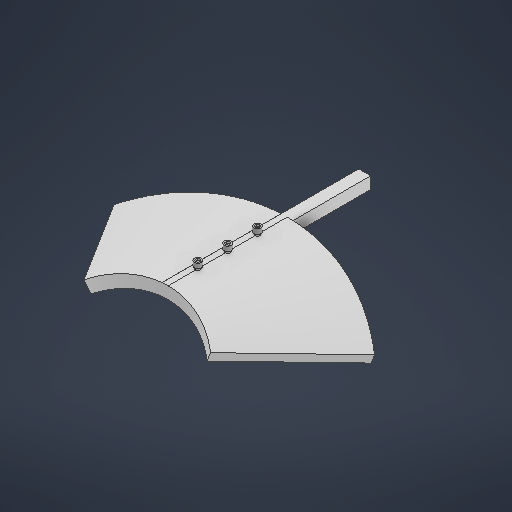
# Autodesk Inventor part: rod
Saved by Autodesk Inventor 2026.2 (Build 302298000, 298)
## iProperties
Created: 2025-12-16
Part Number: rod
Material: Generic
Document SubType Name: Modeling
Designer: Thoma
Density: 1 g/cm^3
Appearance: Default
Author: Thoma
Autodesk Inventor part; units mm, degrees
ref_plane "YZ Plane" through (0, 0, 0) normal (1, 0, 0) x (0, 1, 0)
ref_plane "XZ Plane" through (0, 0, 0) normal (0, 1, 0) x (-1, 0, 0)
ref_plane "XY Plane" through (0, 0, 0) normal (0, 0, 1) x (1, 0, 0)
sketch "Sketch1" plane through (0, 0, 0) normal (0, 1, 0) x (-1, 0, 0)
  line L0 (2.3256, 24.4186) -> (-7.6744, 24.4186)
  line L1 (-7.6744, 24.4186) -> (-7.6744, -75.5814)
  line L2 (-7.6744, -75.5814) -> (2.3256, -75.5814)
  line L3 (2.3256, -75.5814) -> (2.3256, 24.4186)
  point P0 (0, 0)
  dimension "d2" = 100
  dimension "d3" = 10
  constraints: 8 end point, 2 parallel, 1 horizontal, 1 perpendicular
  measures "d2" distance of L2.end L0.start
  measures "d3" distance of L0.start L0.end
extrude "Extrusion1" add sketch "Sketch1" along normal blind 10
sketch "Sketch2" plane through (0, 10, 0) normal (0, 1, 0) x (1, 0, 0)
  line L0 (-2.3256, -24.4186) -> (7.6744, -24.4186) projected
  line L1 (7.6744, -24.4186) -> (7.6744, 75.5814) projected
  line L2 (-2.3256, -24.4186) -> (7.6744, -24.4186)
  line L3 (2.6744, -24.4186) -> (2.6744, -14.4186)
  line L4 (2.6744, -14.4186) -> (2.6744, -4.4186)
  line L5 (2.6744, -4.4186) -> (2.6744, 10.5814)
  line L6 (2.6744, 10.5814) -> (2.6744, 25.5814)
  line L7 (7.6744, 75.5814) -> (-2.3256, 75.5814) projected
  line L8 (-2.3256, 75.5814) -> (7.6744, 75.5814)
  line L9 (2.6744, -24.4186) -> (2.6744, 25.5814)
  line L10 (2.6744, 25.5814) -> (7.6744, 25.5814)
  line L11 (2.6744, 25.5814) -> (-2.3256, 25.5814)
  line L12 (-2.3256, 75.5814) -> (-2.3256, -24.4186) projected
  line L13 (2.6744, 25.5814) -> (2.6744, 40.5814)
  line L14 (2.6744, 25.5814) -> (2.6744, 75.5814)
  line L15 (2.6744, 0.5814) -> (-2.3256, 0.5814)
  line L16 (2.6744, 0.5814) -> (7.6744, 0.5814)
  line L17 (2.6744, 50.5814) -> (-2.3256, 50.5814)
  line L18 (7.6744, 50.5814) -> (2.6744, 50.5814)
  circle A0 centre (2.6744, 0.5814) radius 2
  circle A1 centre (2.6744, 25.5814) radius 2
  circle A2 centre (2.6744, 50.5814) radius 2
  point P0 (0, 0)
  dimension "d28" = 4
  dimension "d29" = 4
  dimension "d30" = 4
  constraints: 30 end point, 6 midpoint, 6 point on line, 5 coincident, 5 vertical, 3 centre point, 2 collinear, 2 perpendicular, 1 horizontal
  measures "d28" diameter of A0
  measures "d29" diameter of A1
  measures "d30" diameter of A2
extrude "Extrusion2" add sketch "Sketch2" along normal blind 2 contours A0 L5 L15 | L15 L5 A0 | A1 L13 L11 | L11 L6 A1 | L16 A0 L5 | L5 A0 L16 | L10 A1 L6 | L13 A1 L10 | A2 L14 L17 | L17 L14 A2 | L18 A2 L14 | L14 A2 L18
sketch "Sketch9" plane through (7.6744, 0, 24.4186) normal (1, 0, 0) x (0, 0, -1)
  line L0 (0, 10) -> (100, 10) projected
  line L1 (0, 0) -> (100, 0) projected
  line L2 (0, 10) -> (100, 10)
  line L3 (100, 10) -> (100, 0)
  line L4 (100, 0) -> (0, 0)
  line L5 (0, 0) -> (0, 10)
  point P0 (24.4186, 0)
  constraints: 8 end point, 2 parallel, 1 horizontal, 1 perpendicular
extrude "Extrusion8" cut sketch "Sketch9" against normal blind 5
sketch "Sketch7" plane through (2.6744, 12, -0.5814) normal (0, 1, 0) x (1, 0, 0)
  arc A0 (0, -2) -> (0, 2) centre (0, 0) ccw projected
  circle A1 centre (0, 0) radius 3
  circle A2 centre (0, 25) radius 3
  arc A3 (0, 48) -> (0, 52) centre (0, 50) ccw projected
  circle A4 centre (0, 50) radius 3
  point P0 (-2.6744, -0.5814)
  dimension "d34" = 6
  dimension "d35" = 6
  dimension "d36" = 6
  constraints: 3 centre point, 2 coincident
  measures "d34" diameter of A4
  measures "d35" diameter of A2
  measures "d36" diameter of A1
extrude "Extrusion6" add sketch "Sketch7" along normal blind 4
sketch "Sketch8" plane through (2.6744, 16, -0.5814) normal (0, 1, 0) x (1, 0, 0)
  line L0 (0, 2) -> (1.7321, 1)
  line L1 (1.7321, 1) -> (1.7321, -1)
  line L2 (1.7321, -1) -> (0, -2)
  line L3 (0, -2) -> (-1.7321, -1)
  line L4 (-1.7321, -1) -> (-1.7321, 1)
  line L5 (-1.7321, 1) -> (0, 2)
  arc A0 (0, 23) -> (0, 27) centre (0, 25) ccw projected
  line L6 (0, 27) -> (1.7321, 26)
  line L7 (1.7321, 26) -> (1.7321, 24)
  line L8 (1.7321, 24) -> (0, 23)
  line L9 (0, 23) -> (-1.7321, 24)
  line L10 (-1.7321, 24) -> (-1.7321, 26)
  line L11 (-1.7321, 26) -> (0, 27)
  arc A1 (0, 48) -> (0, 52) centre (0, 50) ccw projected
  line L12 (0, 52) -> (1.7321, 51)
  line L13 (1.7321, 51) -> (1.7321, 49)
  line L14 (1.7321, 49) -> (0, 48)
  line L15 (0, 48) -> (-1.7321, 49)
  line L16 (-1.7321, 49) -> (-1.7321, 51)
  line L17 (-1.7321, 51) -> (0, 52)
  point P0 (-2.6744, -0.5814)
  point P1 (0, 0)
  point P2 (0, 50)
  dimension "d39" = 2
  constraints: 36 end point, 1 coincident, 1 point on circle, 39 other
  measures "d39" distance of point (0, 0) L0.start
extrude "Extrusion7" cut sketch "Sketch8" against normal blind 1.5 contours L0 L1 L2 L3 L4 L5 | L9 L10 L11 L6 L7 L8 | L15 L16 L17 L12 L13 L14
sketch "Sketch10" plane through (2.6744, 0, 24.4186) normal (1, 0, 0) x (0, 0, -1)
  line L0 (100, 0) -> (100, 10) projected
  line L1 (100, 10) -> (126, 10)
  line L2 (126, 10) -> (126, 29.842)
  line L3 (126, 29.842) -> (100, 10)
  line L4 (126, 29.842) -> (126, 19.842)
  line L5 (126, 19.842) -> (100, 0)
  line L6 (100, 10) -> (165, 10)
  line L7 (165, 10) -> (165, 0)
  line L8 (165, 0) -> (100, 0)
  point P0 (24.4186, 0)
  point P1 (126, 10)
  dimension "d44" = 19.842
  dimension "d45" = 26
  dimension "d46" = 10
  constraints: 16 end point, 3 perpendicular, 2 point on line, 1 horizontal
  measures "d44" distance of L1.end L2.end
  measures "d45" distance of L0.end L1.end
  measures "d46" distance of L2.end L4.end
extrude "Extrusion9" add sketch "Sketch10" against normal blind 5 contours L0 L1 L5 | L5 L1 L6 L7 L8
sketch "Sketch11" plane through (2.6744, 0, 24.4186) normal (1, 0, 0) x (0, 0, -1)
  line L0 (126, 19.842) -> (126, 29.842) projected
  line L1 (126, 19.842) -> (100, 0)
  line L2 (100, 0) -> (-18.0235, -90.0701)
  line L3 (-18.0235, -90.0701) -> (-205.7698, 155.9437)
  line L4 (0, 0) -> (0, 10) projected
  line L5 (0, 9.921) -> (0, 0)
  line L6 (100, 0) -> (0, 0) projected
  line L7 (0, 0) -> (100, 0)
  line L8 (0, 10) -> (23, 10) projected
  line L9 (0, 10) -> (100, 10)
  line L10 (100, 10) -> (126, 29.842)
  line L11 (100, 0) -> (100, 10)
  point P0 (24.4186, 0)
  dimension "d49" = 148.466
  constraints: 16 end point, 3 perpendicular, 1 collinear, 1 horizontal, 1 point on line
  measures "d49" distance of L1.end L2.end
revolve "Revolution2" add sketch "Sketch11" angle 45 about axis through (2.6744, -90.0701, 42.4421) along (0, 0.7949528, 0.6066713) and the other way 45 contours L6 L4 L8 L9 L11
sketch "Sketch12" plane through (2.6744, 0, 24.4186) normal (1, 0, 0) x (0, 0, -1)
  line L0 (100, 0) -> (99.9331, 0) projected
  line L1 (99.9331, 10) -> (99.9331, 0)
  line L2 (165, 0) -> (99.9331, 0) projected
  line L3 (99.9331, 10) -> (165, 10)
  line L4 (165, 10) -> (165, 0)
  line L5 (165, 0) -> (99.9331, 0)
  line L6 (99.9331, 0) -> (99.9331, 10)
  point P0 (24.4186, 0)
  constraints: 10 end point, 2 parallel, 1 horizontal, 1 perpendicular
extrude "Extrusion10" add sketch "Sketch12" along normal blind 5
equation "\"d0\" = d3"
body "Solid1"
